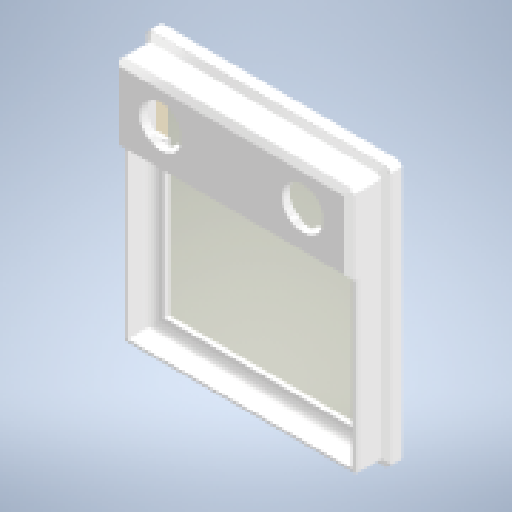
# Autodesk Inventor part: Top
Saved by Autodesk Inventor 2023.1 (Build 271208000, 208)
## iProperties
Created: 2023-03-16
Part Number: Top
Material: PVC, hart
Document SubType Name: Modeling
Designer: nikla
Density: 1.29 g/cm^3
Appearance: Glatt - Weiß
Author: nikla
Autodesk Inventor part; units mm, degrees
ref_plane "YZ Plane" through (0, 0, 0) normal (1, 0, 0) x (0, 1, 0)
ref_plane "XZ Plane" through (0, 0, 0) normal (0, 1, 0) x (-1, 0, 0)
ref_plane "XY Plane" through (0, 0, 0) normal (0, 0, 1) x (1, 0, 0)
sketch "Skizze1" plane through (0, 0, 0) normal (0, 0, 1) x (1, 0, 0)
  line L0 (44.95, -45.95) -> (44.95, 45.95) projected
  line L1 (42.95, 47.95) -> (7.5, 47.95) projected
  line L2 (7.5, 44.95) -> (7.5, 47.95) projected
  line L3 (15, 44.95) -> (7.5, 44.95) projected
  line L4 (15, 44.95) -> (15, 42.95) projected
  line L5 (15, 42.95) -> (39.95, 42.95) projected
  line L6 (39.95, 42.95) -> (39.95, -42.95) projected
  line L7 (39.95, -42.95) -> (-39.95, -42.95) projected
  line L8 (-39.95, -42.95) -> (-39.95, 42.95) projected
  line L9 (-39.95, 42.95) -> (-15, 42.95) projected
  line L10 (-15, 42.95) -> (-15, 44.95) projected
  line L11 (-7.5, 44.95) -> (-15, 44.95) projected
  line L12 (-7.5, 47.95) -> (-7.5, 44.95) projected
  line L13 (-42.95, 47.95) -> (-7.5, 47.95) projected
  line L14 (-44.95, 45.95) -> (-44.95, -45.95) projected
  line L15 (-42.95, -47.95) -> (42.95, -47.95) projected
  line L16 (-44.95, 47.95) -> (44.95, 47.95)
  line L17 (44.95, 47.95) -> (44.95, -47.95)
  line L18 (44.95, -47.95) -> (-44.95, -47.95)
  line L19 (-44.95, -47.95) -> (-44.95, 47.95)
  line L20 (-15, 42.95) -> (-15, 36.95)
  line L21 (-15, 36.95) -> (-39.95, 36.95)
  line L22 (0, -67.13) -> (0, 67.13) projected
  line L23 (15, 42.95) -> (15, 36.95)
  line L24 (15, 36.95) -> (39.95, 36.95)
  line L25 (-39.95, -39.95) -> (-39.95, 36.95)
  line L26 (36.95, -42.95) -> (-36.95, -42.95)
  line L27 (-15, 42.95) -> (15, 42.95)
  line L28 (39.95, 36.95) -> (39.95, -39.95)
  line L29 (39.95, -39.95) -> (39.95, -42.95)
  line L30 (36.95, -42.95) -> (39.95, -42.95)
  line L31 (-36.95, -42.95) -> (-39.95, -42.95)
  line L32 (-39.95, -39.95) -> (-39.95, -42.95)
  point P0 (0, 0)
  point P1 (-15, 43.95)
  point P2 (-15, 39.95)
  constraints: 34 end point, 5 symmetric about line, 4 collinear, 4 parallel, 2 horizontal, 2 midpoint, 2 perpendicular, 1 vertical alignment
extrude "Extrusion1" add sketch "Skizze1" along normal blind 1 contours L20 L21 L8 L9 | L5 L6 L24 L23
sketch "Skizze2" plane through (0, 0, 1) normal (0, 0, 1) x (1, 0, 0)
  line L0 (44.95, -45.95) -> (44.95, 45.95) projected
  line L1 (-44.95, -47.95) -> (44.95, -47.95)
  line L2 (44.95, -47.95) -> (44.95, 47.95)
  line L3 (44.95, 47.95) -> (-44.95, 47.95)
  line L4 (-44.95, 47.95) -> (-44.95, -47.95)
  line L5 (-42.95, -45.95) -> (42.95, -45.95)
  line L6 (42.95, -45.95) -> (42.95, 45.95)
  line L7 (42.95, 45.95) -> (-42.95, 45.95)
  line L8 (-42.95, 45.95) -> (-42.95, -45.95)
  point P0 (0, 0)
  point P1 (44.95, -47.95)
  point P2 (44.95, -47.95)
  point P3 (44.95, -44.95)
  point P4 (44.95, 44.95)
  point P5 (44.95, -44.95)
  point P6 (44.95, 44.95)
  dimension "d5" = 2
  dimension "d6" = 2
  dimension "d7" = 2
  dimension "d8" = 2
  constraints: 16 end point, 4 parallel, 2 horizontal, 2 perpendicular
  measures "d5" distance between parallel lines of L1 L5
  measures "d6" distance between parallel lines of L3 L7
  measures "d7" distance between parallel lines of L4 L8
  measures "d8" distance between parallel lines of L0 L6
extrude "Extrusion2" add sketch "Skizze2" along normal blind 10
sketch "Skizze3" plane through (0, 0, 11) normal (0, 0, 1) x (1, 0, 0)
  line L0 (44.95, -45.95) -> (44.95, 45.95) projected
  line L1 (-44.95, 45.95) -> (-44.95, -45.95) projected
  line L2 (44.95, 47.95) -> (-44.95, 47.95)
  line L3 (-44.95, 47.95) -> (-44.95, 17.95)
  line L4 (-44.95, 17.95) -> (44.95, 17.95)
  line L5 (44.95, 17.95) -> (44.95, 47.95)
  circle A0 centre (27.1853, 34.028) radius 1.75
  circle A1 centre (-27.25, 34.028) radius 1.75 projected
  circle A2 centre (-27.25, 34.028) radius 8
  circle A3 centre (27.1853, 34.028) radius 8
  point P0 (0, 0)
  point P1 (44.95, -47.95)
  point P2 (-44.95, 47.95)
  point P3 (-44.95, -47.95)
  point P4 (-44.95, 47.95)
  point P5 (44.95, 17.95)
  point P6 (44.95, -44.95)
  point P7 (44.95, 44.95)
  point P8 (-44.95, 44.95)
  point P9 (-44.95, -44.95)
  point P10 (-44.95, 44.95)
  point P11 (44.95, 17.95)
  dimension "d11" = 30
  dimension "d12" = 16
  dimension "d13" = 16
  constraints: 8 end point, 3 centre point, 2 coincident, 2 parallel, 1 horizontal, 1 horizontal alignment, 1 perpendicular, 1 point on line
  measures "d11" distance of L3.end L2.end
  measures "d12" diameter of A2
  measures "d13" diameter of A3
extrude "Extrusion3" add sketch "Skizze3" along normal blind 3 contours L4 L1 L3 L2 L5 L0
fillet "Rundung2" [suppressed]
fillet "Rundung3" [suppressed]
sketch "Skizze4" plane through (0, 0, 1) normal (0, 0, -1) x (-1, 0, 0)
  line L0 (-44.95, 47.95) -> (44.95, 47.95) projected
  line L1 (42.95, 45.95) -> (-42.95, 45.95) projected
  line L2 (7.5, 45.95) -> (-7.5, 45.95)
  line L3 (-7.5, 45.95) -> (-7.5, 47.95)
  line L4 (-7.5, 47.95) -> (7.5, 47.95)
  line L5 (7.5, 47.95) -> (7.5, 45.95)
  line L6 (-44.95, -47.95) -> (-44.95, 47.95) projected
  line L7 (44.95, -47.95) -> (-44.95, -47.95) projected
  line L8 (44.95, 47.95) -> (44.95, -47.95) projected
  line L9 (42.95, -45.95) -> (42.95, 45.95) projected
  line L10 (-42.95, -45.95) -> (42.95, -45.95) projected
  line L11 (-42.95, 45.95) -> (-42.95, -45.95) projected
  point P0 (0, 0)
  constraints: 8 end point, 2 parallel, 1 horizontal, 1 perpendicular
extrude "Extrusion4" add sketch "Skizze4" along normal blind 5.5 contours L0 L3 L1 L11 L10 L9 L5 L8 L7 L6 | L0 L5 L1 L3
chamfer "Fase1" distance 1 angle 45 3 edges at (-44.95, -15, 11) (0, -47.95, 11) (44.95, -15, 11)
sketch "Skizze5" plane through (0, 0, 11) normal (0, 0, -1) x (-1, 0, 0)
  circle A0 centre (26.75, 21.7) radius 1.1 projected
  circle A1 centre (-27.25, 21.65) radius 1.1 projected
  circle A2 centre (26.75, 21.7) radius 2.75
  circle A3 centre (-27.25, 21.65) radius 2.75
  circle A4 centre (26.75, 21.7) radius 0.9
  circle A5 centre (-27.25, 21.65) radius 0.9
  point P0 (0, 0)
  dimension "d24" = 5.5
  dimension "d25" = 5.5
  dimension "d26" = 1.8
  dimension "d27" = 1.8
  constraints: 4 centre point, 4 coincident
  measures "d24" diameter of A2
  measures "d25" diameter of A3
  measures "d26" diameter of A4
  measures "d27" diameter of A5
extrude "Extrusion5" add sketch "Skizze5" along normal blind 4 contours A0 | A1 | A2 | A3
chamfer "Fase2" distance 2 angle 45 4 edges at (-44.95, 32.95, 14) (0, 47.95, 14) (0, 17.95, 14) (44.95, 32.95, 14)
sketch "Skizze6" plane through (0, 0, 1) normal (0, 0, 1) x (1, 0, 0)
  line L0 (-42.95, -45.95) -> (-42.95, 17.95) projected
  line L1 (42.95, -45.95) -> (-42.95, -45.95) projected
  line L2 (42.95, 17.95) -> (42.95, -45.95) projected
  line L3 (-7.5, 45.95) -> (-42.95, 45.95) projected
  line L4 (-42.95, 45.95) -> (-42.95, -45.95) projected
  line L5 (42.95, -45.95) -> (42.95, 45.95) projected
  line L6 (-42.95, 13.95) -> (-39.95, 13.95)
  line L7 (-39.95, 42.95) -> (-39.95, 36.95) projected
  line L8 (-39.95, 13.95) -> (-39.95, 36.95)
  line L9 (-39.95, 36.95) -> (-15, 36.95) projected
  line L10 (-39.95, 36.95) -> (-15, 36.95)
  line L11 (-39.95, 13.95) -> (-39.95, 36.95)
  line L12 (-15, 36.95) -> (-15, 44.95) projected
  line L13 (-15, 36.95) -> (-15, 44.95)
  line L14 (-15, 44.95) -> (0, 44.95)
  line L15 (0, -64.33) -> (0, 64.33) projected
  line L16 (42.95, 13.95) -> (39.95, 13.95)
  line L17 (39.95, 13.95) -> (39.95, 36.95)
  line L18 (39.95, 36.95) -> (15, 36.95)
  line L19 (15, 36.95) -> (15, 44.95)
  line L20 (15, 44.95) -> (0, 44.95)
  line L21 (-42.95, 13.95) -> (-42.95, 45.95)
  line L22 (42.95, 45.95) -> (-42.95, 45.95) projected
  line L23 (0, 45.95) -> (-42.95, 45.95)
  line L24 (0, 45.95) -> (42.95, 45.95)
  line L25 (42.95, 13.95) -> (42.95, 45.95)
  point P0 (0, 0)
  point P1 (-39.95, -42.95)
  point P2 (7.5, 45.95)
  point P3 (7.5, 45.95)
  dimension "d36" = 32
  constraints: 30 end point, 5 symmetric about line, 4 collinear, 2 perpendicular, 2 point on line, 2 vertical, 1 horizontal, 1 midpoint, 1 vertical alignment
  measures "d36" distance between parallel lines of L3 L6
extrude "Extrusion6" cut sketch "Skizze6" against normal blind 10 contours L0 L4 L3 L22 L15 L14 L12 L9 L8 L6 | L15 L22 L5 L2 L16 L17 L18 L19 L20
sketch "Skizze7" plane through (0, 0, 0) normal (0, 0, -1) x (-1, 0, 0)
  line L0 (-44.95, -47.95) -> (-44.95, 17.95) projected
  line L1 (44.95, 47.95) -> (-44.95, 47.95)
  line L2 (-44.95, 47.95) -> (-44.95, -47.95)
  line L3 (-44.95, -47.95) -> (44.95, -47.95)
  line L4 (44.95, -47.95) -> (44.95, 47.95)
  line L5 (44.95, 47.95) -> (-44.95, -47.95) construction
  line L6 (-44.95, 47.95) -> (44.95, -47.95) construction
  line L7 (46.8249, 49.95) -> (-46.8249, 49.95)
  line L8 (-46.8249, 49.95) -> (-46.8249, -49.95)
  line L9 (-46.8249, -49.95) -> (46.8249, -49.95)
  line L10 (46.8249, -49.95) -> (46.8249, 49.95)
  line L11 (46.8249, 49.95) -> (-46.8249, -49.95) construction
  line L12 (-46.8249, 49.95) -> (46.8249, -49.95) construction
  point P0 (0, 0)
  point P1 (-44.95, 17.95)
  dimension "d42" = 2
  constraints: 24 end point, 4 midpoint, 4 parallel, 2 horizontal, 2 perpendicular, 1 point on line
  measures "d42" distance between parallel lines of L3 L9
extrude "Extrusion7" add sketch "Skizze7" along normal up to surface (4.5 mm away)
chamfer "Fase5" distance 1.87 angle 45 4 edges at (44.95, 0, 0) (0, 47.95, 0) (-44.95, 0, 0) (0, -47.95, 0)
chamfer "Fase6" distance 1.5 angle 45 12 edges at (-46.8249, -49.95, -2.25) (-45.885, -48.885, 0.935) (-44.95, -47.95, 5.935) (44.95, -47.95, 5.935) (45.885, -48.885, 0.935) (46.8249, -49.95, -2.25) (44.95, 47.95, 6.935) (45.885, 48.885, 0.935) (46.8249, 49.95, -2.25) (-44.95, 47.95, 6.935) (-45.885, 48.885, 0.935) (-46.8249, 49.95, -2.25)
ref_plane "Arbeitsebene1" through (0, 0, 0) normal (0, 0, 1) x (1, 0, 0)
sketch "Skizze8" plane through (0, 0, 0) normal (0, 0, 1) x (1, 0, 0)
  line L0 (-42.95, -45.95) -> (-42.95, 17.95) projected
  line L1 (42.95, -45.95) -> (-42.95, -45.95) projected
  line L2 (42.95, 17.95) -> (42.95, -45.95) projected
  line L3 (-42.95, 17.95) -> (-37.95, 17.95)
  line L4 (-42.95, 45.95) -> (-42.95, -45.95) projected
  line L5 (-42.95, 17.95) -> (-37.95, 17.95) construction
  line L6 (-37.95, 17.95) -> (-37.95, -40.95)
  line L7 (-37.95, -40.95) -> (0, -40.95)
  line L8 (0, -67.13) -> (0, 67.13)
  line L9 (42.95, 17.95) -> (37.95, 17.95)
  line L10 (37.95, 17.95) -> (37.95, -40.95)
  line L11 (37.95, -40.95) -> (0, -40.95)
  point P0 (0, 0)
  point P1 (0, 0)
  dimension "d51" = 5
  dimension "d52" = 0
  dimension "d54" = 5
  constraints: 16 end point, 2 perpendicular, 2 symmetric about line, 1 collinear, 1 horizontal, 1 midpoint, 1 vertical, 1 vertical alignment, 2 other
  measures "d51" distance of L0.end L3.end
  measures "d52" distance between parallel lines of L3 L5
  measures "d54" distance between parallel lines of L1 L7
extrude "Extrusion8" add sketch "Skizze8" along normal blind 2
fillet "Rundung4" radius 3.75 3 edges at (-42.95, -14, 2) (0, -45.95, 2) (42.95, -14, 2)
